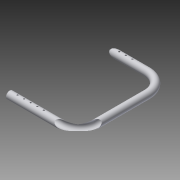
# Autodesk Inventor part: Rura_pionowa_podnóżka
Saved by Autodesk Inventor 2015 (Build 190159000, 159)
## iProperties
Created: 2015-12-07
Part Number: Rura_pionowa_podnóżka
Material: Aluminium AW-7020
Document SubType Name: Modeling
Designer: graaapsik
Density: 2.78 g/cm^3
Appearance: Aluminium AW-7020
Mass: 272.705 g
Surface Area: 1316.06 cm^2
Volume: 98.0953 cm^3
Author: graaapsik
Autodesk Inventor part; units mm, degrees
ref_plane "Płaszczyzna konstrukcyjna1" through (0, 0, 0) normal (0, 0, 1) x (1, 0, 0)
sketch "Szkic1" plane through (0, 0, 0) normal (0, 0, 1) x (1, 0, 0)
  line L0 (-242.565, 352.7157) -> (0, 352.7157) construction
  ellipse E0 centre (0, 336.7157) end of major axis (0, 320.7157) minor radius 0 construction
  line L1 (0, 336.7157) -> (-4.551, 336.7157) construction
  line L2 (0, 336.7157) -> (185, 336.7157)
  line L3 (260, 261.7157) -> (260, 75)
  line L4 (185, 0) -> (0, 0)
  arc A0 (260, 261.7157) -> (185, 336.7157) centre (185, 261.7157) ccw
  arc A1 (185, 0) -> (260, 75) centre (185, 75) ccw
  dimension "d0" = 260
  dimension "d1" = 75
  constraints: 10 end point, 4 point on circle, 4 tangent, 3 horizontal, 2 centre point, 1 collinear, 1 equal radius, 1 vertical, 3 other
  measures "d0" distance from line of L3 L4.end
  measures "d1" radius of A0
ref_plane "Płaszczyzna konstrukcyjna2" through (0, 336.7157, 0) normal (1, 0, 0) x (0, 0.0872, -0.9962)
sketch "Szkic2" plane through (0, 336.7157, 0) normal (1, 0, 0) x (0, 0.0872, -0.9962)
  circle A0 centre (0, 0) radius 14 projected
  circle A1 centre (0, 0) radius 14
  circle A2 centre (0, 0) radius 12.5
  point P0 (-29.3467, -335.4344)
  dimension "d2" = 1.5
  constraints: 2 centre point, 1 coincident, 1 concentric
  measures "d2" radial gap between concentric circles of A2 A0
sweep "Przeciągnięcie1" add profiles "Szkic2" path "Szkic1"
ref_plane "Płaszczyzna konstrukcyjna3" through (0, 0, 14) normal (0, 0, 1) x (1, 0, 0)
sketch "Szkic3" plane through (0, 0, 14) normal (0, 0, 1) x (1, 0, 0)
  line L0 (273.78, 176.3063) -> (25.8333, 176.3063) construction
  line L1 (184.2429, 354.0551) -> (184.296, 352.8395) projected
  line L2 (184.296, 352.8395) -> (184.2429, 354.0551) projected
  ellipse E0 centre (-1.175, 336.6129) end of major axis (-1.175, 350.6129) minor radius 0 construction
  line L3 (260, 261.7157) -> (260, 75) projected
  line L4 (260, 168.3579) -> (-77.8228, 168.3579) construction
  line L5 (185, 0) -> (0, 0) projected
  arc A0 (185, 0) -> (260, 75) centre (185, 75) ccw projected
  arc A1 (260, 261.7157) -> (185, 336.7157) centre (185, 261.7157) ccw projected
  line L6 (0, 336.7157) -> (185, 336.7157) projected
  ellipse E1 centre (0, 0) end of major axis (0, 14) minor radius 0 projected
  ellipse E2 centre (0, 336.7157) end of major axis (0, 350.7157) minor radius 0 projected
  point P0 (30, 336.7157)
  point P1 (55, 336.7157)
  point P2 (80, 336.7157)
  point P3 (105, 336.7157)
  point P4 (130, 336.7157)
  point P5 (-1.2947, 0.1133)
  point P6 (30, 0)
  point P7 (55, 0)
  point P8 (80, 0)
  point P9 (105, 0)
  point P10 (130, 0)
  dimension "d3" = 0
  dimension "d7" = 25
  dimension "d32" = 25
  dimension "d37" = 25
  dimension "d38" = 30
  dimension "d39" = 25
  dimension "d40" = 25
  dimension "d41" = 30
  constraints: 8 point on line, 4 end point, 2 coincident, 1 horizontal, 1 midpoint, 1 perpendicular, 5 other
  measures "d7" distance of point (30, 336.716) point (55, 336.716)
  measures "d32" distance of point (30, 0) point (55, 0)
  measures "d37" distance of point (105, 0) point (130, 0)
  measures "d38" distance of point (0, 0) point (30, 0)
  measures "d39" distance of point (55, 0) point (80, 0)
  measures "d40" distance of point (105, 0) point (80, 0)
  measures "d41" distance of point (0, 336.716) point (30, 336.716)
hole "Otwór1" at (30, 336.7157, 14) at (55, 336.7157, 14) at (80, 336.7157, 14) at (105, 336.7157, 14) at (130, 336.7157, 14) at (30, 0, 14) at (55, 0, 14) at (80, 0, 14) at (105, 0, 14) at (130, 0, 14) direction (0, 0, -1) diameter 6 end through all
ref_plane "Płaszczyzna konstrukcyjna4" through (246, 0, 0) normal (1, 0, 0) x (0, 1, 0)
ref_plane "Płaszczyzna konstrukcyjna5" through (0, 0, -14) normal (0, 0, 1) x (1, 0, 0)
